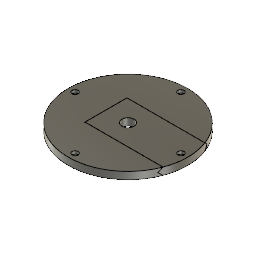
bottomplate (Autodesk Fusion 360 design; units mm, degrees)
Autodesk Fusion 360 part; units mm, degrees
note: some values were not read from the file. Chosen so that the rebuilt part matches the saved one: which bodies a step acts on. Set by a fixed rule: which face or edge a step refers to.
sketch "Skizze1" plane through (0, 0, 0) normal (0, 0, 1) x (1, 0, 0)
  circle A0 centre (0, 0) radius 57
  line L0 (-100, 0) -> (100, 0) construction
  line L1 (0, 100) -> (0, -100) construction
  circle A1 centre (50.5, 0) radius 2.45
  line L2 (-57, 57) -> (57, 57) construction
  line L3 (57, 57) -> (57, -57) construction
  line L4 (57, -57) -> (-57, -57) construction
  line L5 (-57, -57) -> (-57, 57) construction
  circle A2 centre (-50.5, 0) radius 2.45
  circle A3 centre (0, 50.5) radius 2.45
  circle A4 centre (0, -50.5) radius 2.45
  circle A5 centre (50.5, 0) radius 4.75
  circle A6 centre (0, 50.5) radius 4.75
  circle A7 centre (-50.5, 0) radius 4.75
  circle A8 centre (0, -50.5) radius 4.75
  dimension "d1" = 114
  dimension "d2" = 4.9
  dimension "d3" = 6.5
  dimension "d4" = 4.9
  dimension "d5" = 6.5
  dimension "d6" = 4.9
  dimension "d7" = 4.9
  dimension "d8" = 6.5
  dimension "d9" = 6.5
  dimension "d10" = 9.5
  dimension "d11" = 9.5
  dimension "d12" = 9.5
  dimension "d13" = 9.5
  measures "d1" diameter of A0
  measures "d2" diameter of A1
  measures "d4" diameter of A2
  measures "d6" diameter of A3
  measures "d7" diameter of A4
  measures "d10" diameter of A5
  measures "d11" diameter of A6
  measures "d12" diameter of A7
  measures "d13" diameter of A8
extrude "Extrusion1" add sketch "Skizze1" against normal blind 1.8 contours A5 | A6 | A7 | A8 makes body 1 at (4.7264, -50.9729, -0.6) makes body 2 at (-45.7736, -0.4729, -0.6) makes body 3 at (55.2264, -0.4729, -0.6) makes body 4 at (4.7264, 50.0271, -0.6)
chamfer "Fase1" distance 2.3 distance2 1.8 4 edges at (-54.9286, 1.7177, -1.8) (-4.4286, 52.2177, -1.8) (46.0714, 1.7177, -1.8) (-4.4286, -48.7823, -1.8) measured on face at (-46.5435, -0.3577, -1.8) measured on face at (3.9565, 50.1423, -1.8) measured on face at (54.4565, -0.3577, -1.8) measured on face at (3.9565, -50.8577, -1.8) on bodies 1 2 3 4
extrude "Extrusion2" add sketch "Skizze1" against normal blind 1.5 contours A1 | A2 | A3 | A4 bodies 1 2 3 4
extrude "Extrusion3" add sketch "Skizze1" along normal blind 7 contours A0 | A1 | A2 | A3 | A4 | A5 | A6 | A7 | A8 bodies 1 2 3 4
sketch "Skizze2" plane through (0, 0, 7) normal (0, 0, 1) x (-1, 0, 0)
  circle A0 centre (0, 0) radius 57
  circle A1 centre (-50.5, 0) radius 1.45
  circle A2 centre (50.5, 0) radius 1.45
  circle A3 centre (0, 50.5) radius 1.45
  circle A4 centre (0, -50.5) radius 1.45
  circle A5 centre (-50.5, 0) radius 2.9
  circle A6 centre (0, -50.5) radius 2.9
  circle A7 centre (50.5, 0) radius 2.9
  circle A8 centre (0, 50.5) radius 2.9
  dimension "d22" = 2.9
  dimension "d23" = 2.9
  dimension "d24" = 2.9
  dimension "d25" = 2.9
  dimension "d28" = 5.8
  dimension "d29" = 5.8
  dimension "d30" = 5.8
  dimension "d31" = 5.8
  measures "d22" diameter of A1
  measures "d23" diameter of A2
  measures "d24" diameter of A3
  measures "d25" diameter of A4
  measures "d28" diameter of A5
  measures "d29" diameter of A6
  measures "d30" diameter of A7
  measures "d31" diameter of A8
extrude "Extrusion5" cut sketch "Skizze2" against normal blind 2.8 contours A5 | A6 | A7 | A8 bodies 1
extrude "Extrusion4" cut sketch "Skizze2" against normal up to surface (8.5 mm away) contours A1 | A2 | A3 | A4 bodies 1
sketch "Skizze3" plane through (0, 0, 7) normal (0, 0, 1) x (-1, 0, 0)
  circle A0 centre (0, 50.5) radius 2.9
  circle A1 centre (50.5, 0) radius 2.9
  circle A2 centre (-50.5, 0) radius 2.9
  circle A3 centre (0, -50.5) radius 2.9
  circle A4 centre (0, 0) radius 57
  circle A5 centre (0, 0) radius 5.8
  dimension "d34" = 11.6
  measures "d34" diameter of A5
extrude "Extrusion6" cut sketch "Skizze3" against normal blind 7 contours A5 bodies 1
chamfer "Fase2" distance 0.4 distance2 1.4 4 edges at (51.8519, 0.5243, 4.2) (1.3519, -49.9757, 4.2) (-49.1481, 0.5243, 4.2) (1.3519, 51.0243, 4.2) measured on face at (50.2482, -1.428, 2.3) measured on face at (-1.4428, -50.3556, 2.3) measured on face at (-50.7518, -1.428, 2.3) measured on face at (1.4052, 50.1422, 0.4) on bodies 1
sketch "Skizze4" plane through (0, 0, 0) normal (1, 0, 0) x (0, 1, 0)
  line L0 (57, 7) -> (-57, 7)
  line L1 (20, 7) -> (23.5, 3.5)
  line L2 (57, 0) -> (-57, 0)
  line L3 (23.5, 3.5) -> (20, 0)
  line L4 (20, 7) -> (20, 0) construction
  line L5 (20, 3.5) -> (23.5, 3.5) construction
  line L6 (0, 0) -> (0, 7) construction
  line L7 (-23.5, 3.5) -> (-20, 0)
  line L8 (-20, 7) -> (-23.5, 3.5)
  dimension "d41" = 45
  dimension "d42" = 20
  measures "d41" angle of L1 L4
  measures "d42" distance of L6.start L4
surface "Extrusion7" add extruded along (1, 0, 0) between -71 and 71 path "Skizze4" along L8 L7 L1 L3 separate body makes body 5 at (23.6667, -22.3333, 2.3333) makes body 6 at (23.6667, 22.3333, 2.3333)
split "Teilen1" by bodies 6 bodies 1 makes body 7 at (-0.0722, 29.2027, 7)
split "Teilen2" by bodies 5 bodies 1 makes body 8 at (-0.0722, -29.2027, 7)
move_body "Verschieben1" bodies 6 to x (0, 1, 0) y (-1, 0, 0) z (0, 0, 1) at (-1, 1, 0)
split "Teilen3" by bodies 6 bodies 1 makes body 9 at (-29.8667, 0, 7)
delete_body "Körper entfernen1" bodies 6
delete_body "Körper entfernen2" bodies 5
combine "Kombinieren1" operation add target body 7 tool bodies 9 8
equation "d4 = d2"
equation "d5 = d3"
equation "d6 = d2"
equation "d7 = d2"
equation "d8 = d3"
equation "d9 = d3"
